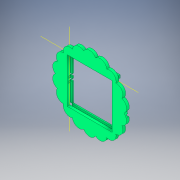
# Autodesk Inventor part: 20_Cube_Insert_CirAp_Wheel
Saved by Autodesk Inventor 2019.4 (Build 234330000, 330)
## iProperties
Created: 2019-10-23
Part Number: 20_Cube_Insert_CirAp_Wheel
Material: Generic
Document SubType Name: Modeling
Designer: marsikovabarbora
Density: 1 g/cm^3
Appearance: Default
Author: marsikovabarbora
Autodesk Inventor part; units mm, degrees
note: some values were not read from the file. Chosen so that the rebuilt part matches the saved one: copy form of "Mirror1".
ref_plane "Work Plane1" through (0, 0, 0) normal (0, 0, 1) x (1, 0, 0)
sketch "Sketch1" plane through (0, 0, 0) normal (0, 0, 1) x (1, 0, 0)
  circle A0 centre (0, 0) radius 20 construction
  line L0 (24.9006, -16.8) -> (24.9006, 16.8) construction
  line L1 (24.9006, 16.8) -> (21.2406, 16.8) construction
  line L2 (21.2406, 16.8) -> (16.8, 21.2406) construction
  line L3 (16.8, 21.2406) -> (16.8, 24.9006) construction
  line L4 (16.8, 24.9006) -> (-16.8, 24.9006) construction
  line L5 (-16.8, 24.9006) -> (-16.8, 21.2406) construction
  line L6 (-16.8, 21.2406) -> (-21.2406, 16.8) construction
  line L7 (-21.2406, 16.8) -> (-24.9006, 16.8) construction
  line L8 (-24.9006, 16.8) -> (-24.9006, -16.8) construction
  line L9 (-24.9006, -16.8) -> (-21.2406, -16.8) construction
  line L10 (-21.2406, -16.8) -> (-16.8, -21.2406) construction
  line L11 (-16.8, -21.2406) -> (-16.8, -24.9006) construction
  line L12 (-16.8, -24.9006) -> (16.8, -24.9006) construction
  line L13 (16.8, -24.9006) -> (16.8, -21.2406) construction
  line L14 (16.8, -21.2406) -> (21.2406, -16.8) construction
  line L15 (21.2406, -16.8) -> (24.9006, -16.8) construction
  line L16 (-36.8547, 0) -> (36.8547, 0) construction
  line L17 (0, -36.4) -> (0, 36.4) construction
  circle A1 centre (0, 0) radius 26
  circle A2 centre (0, 0) radius 22
  point P0 (0, 0)
  dimension "d0" = 52
  dimension "d1" = 44
  constraints: 2 centre point, 2 coincident
  measures "d0" diameter of A1
  measures "d1" diameter of A2
extrude "Extrusion1" add sketch "Sketch1" along normal blind 1.9
sketch "Sketch2" plane through (0, 0, 1.9) normal (0, 0, 1) x (1, 0, 0)
  circle A0 centre (0, 0) radius 22 construction
  circle A1 centre (0, 0) radius 26 construction
  line L0 (0, -36.4197) -> (0, 36.5183) construction
  line L1 (0, 0) -> (-4.5149, 25.605) construction
  line L2 (0, 0) -> (4.5149, 25.605) construction
  arc A2 (0, 26) -> (-4.5149, 25.605) centre (0, 0) ccw
  arc A3 (4.5149, 25.605) -> (0, 26) centre (0, 0) ccw
  arc A4 (4.1452, 23.5087) -> (-4.1452, 23.5087) centre (0, 21.3057) ccw
  line L3 (-4.1452, 23.5087) -> (0, 22) construction
  line L4 (4.1452, 23.5087) -> (0, 22) construction
  line L5 (-4.5149, 25.605) -> (-4.1452, 23.5087)
  line L6 (4.5149, 25.605) -> (4.1452, 23.5087)
  point P0 (0, 26)
  dimension "d62" = 10
  dimension "d63" = 10
  dimension "d65" = 70
  dimension "d66" = 70
  constraints: 12 end point, 8 point on circle, 4 point on line, 3 centre point, 2 collinear, 2 vertical alignment, 1 coincident
  measures "d62" angle of L1 L0
  measures "d63" angle of L2 L0
  measures "d65" angle of L4 L0
  measures "d66" angle of L0 L3
extrude "Extrusion2" cut sketch "Sketch2" against normal up to next
mirror "Mirror1" about plane through (0, 0, 0) normal (1, 0, 0) of "Extrusion2" geometry pattern yes
pattern_circular "Circular Pattern1" count 18 over 360 about axis through (0, 0, -10) along (0, 0, 1) of "Extrusion2", "Mirror1"
sketch "Skizze4" plane through (0, 0, 1.9) normal (0, 0, 1) x (1, 0, 0)
  circle A0 centre (0, 0) radius 22 projected
  line L0 (15.5563, 15.5563) -> (15.5563, -15.5563)
  line L1 (15.5563, -15.5563) -> (-15.5563, -15.5563)
  line L2 (-15.5563, -15.5563) -> (-15.5563, 15.5563)
  line L3 (-15.5563, 15.5563) -> (15.5563, 15.5563)
  arc A1 (-15.5563, 15.5563) -> (-15.5563, -15.5563) centre (0, 0) ccw
  arc A2 (15.5563, 15.5563) -> (-15.5563, 15.5563) centre (0, 0) ccw
  arc A3 (15.5563, -15.5563) -> (15.5563, 15.5563) centre (0, 0) ccw
  arc A4 (-15.5563, -15.5563) -> (15.5563, -15.5563) centre (0, 0) ccw
  point P0 (-15.5563, 0)
  constraints: 8 end point, 8 point on circle, 4 centre point, 2 coincident, 1 horizontal alignment, 1 midpoint, 12 other
extrude "Extrusion4" add sketch "Skizze4" against normal up to surface (1.9 mm away) contours A0 L0 | L3 A0 | A0 L1 | L2 A0
sketch "Skizze5" plane through (0, 0, 0) normal (0, 0, -1) x (-1, 0, 0)
  line L0 (17, 17) -> (17, 15.2314)
  line L1 (17, -17) -> (-17, -17)
  line L2 (-17, -17) -> (-17, 17)
  line L3 (-17, 17) -> (14.1379, 17)
  line L4 (11.6421, 17) -> (14.0421, 17)
  line L5 (17, 15.2314) -> (17, -17)
  line L6 (15.2175, 17) -> (17, 17)
  line L7 (14.1379, 17) -> (15.2175, 17)
  line L8 (15.5563, -15.5563) -> (15.5563, 15.5563) projected
  line L9 (15.5563, 15.5563) -> (-15.5563, 15.5563) projected
  line L10 (-15.5563, 15.5563) -> (-15.5563, -15.5563) projected
  line L11 (-15.5563, -15.5563) -> (15.5563, -15.5563) projected
  arc A0 (-4.1452, 23.5087) -> (-11.9357, 20.6732) centre (-7.287, 20.0208) ccw projected
  arc A1 (4.1452, 23.5087) -> (-4.1452, 23.5087) centre (0, 21.3057) ccw projected
  arc A2 (11.9357, 20.6732) -> (4.1452, 23.5087) centre (7.287, 20.0208) ccw projected
  arc A3 (18.2866, 15.3442) -> (11.9357, 20.6732) centre (13.6951, 16.3211) ccw projected
  arc A4 (22.4318, 8.1645) -> (18.2866, 15.3442) centre (18.4513, 10.6529) ccw projected
  arc A5 (23.8714, 0) -> (22.4318, 8.1645) centre (20.9821, 3.6997) ccw projected
  arc A6 (22.4318, -8.1645) -> (23.8714, 0) centre (20.9821, -3.6997) ccw projected
  arc A7 (18.2866, -15.3442) -> (22.4318, -8.1645) centre (18.4513, -10.6529) ccw projected
  arc A8 (11.9357, -20.6732) -> (18.2866, -15.3442) centre (13.6951, -16.3211) ccw projected
  arc A9 (4.1452, -23.5087) -> (11.9357, -20.6732) centre (7.287, -20.0208) ccw projected
  arc A10 (-4.1452, -23.5087) -> (4.1452, -23.5087) centre (0, -21.3057) ccw projected
  arc A11 (-11.9357, -20.6732) -> (-4.1452, -23.5087) centre (-7.287, -20.0208) ccw projected
  arc A12 (-18.2866, -15.3442) -> (-11.9357, -20.6732) centre (-13.6951, -16.3211) ccw projected
  arc A13 (-22.4318, -8.1645) -> (-18.2866, -15.3442) centre (-18.4513, -10.6529) ccw projected
  arc A14 (-23.8714, 0) -> (-22.4318, -8.1645) centre (-20.9821, -3.6997) ccw projected
  arc A15 (-22.4318, 8.1645) -> (-23.8714, 0) centre (-20.9821, 3.6997) ccw projected
  arc A16 (-18.2866, 15.3442) -> (-22.4318, 8.1645) centre (-18.4513, 10.6529) ccw projected
  arc A17 (-11.9357, 20.6732) -> (-18.2866, 15.3442) centre (-13.6951, 16.3211) ccw projected
  point P0 (0, 0)
  point P1 (0, 0)
  point P2 (0, 17)
  dimension "d26" = 34
  constraints: 16 end point, 2 point on line, 1 coincident, 1 collinear, 1 vertical alignment, 9 other
  measures "d26" distance of L2.end L0.start
ref_plane "Arbeitsebene2" through (7.7782, 15.5563, 0) normal (0, 1, 0) x (1, 0, 0)
sketch "Skizze6" plane through (7.7782, 15.5563, 0) normal (0, 1, 0) x (1, 0, 0)
  line L0 (-26.9158, 0) -> (-26.9158, 0) projected
  line L1 (15.5563, 15.5563) -> (-15.5563, 15.5563)
  line L2 (-23.3345, 0) -> (7.7782, 0) projected
  line L3 (-24.7782, 0) -> (-25.7782, 0)
  line L4 (-24.7782, 1.5) -> (-24.7782, 0)
  line L5 (-24.7782, 19.0476) -> (-24.7782, -5.3913) projected
  line L6 (-23.3345, 0) -> (-27.3072, 0)
  line L7 (-24.7782, 1.5) -> (-23.3782, 1.5)
  line L8 (-23.3782, 1.5) -> (-23.3782, 2.5)
  line L9 (-23.3782, 2.5) -> (-25.2782, 2.5)
  line L10 (-25.2782, 2.5) -> (-25.7782, 0)
  point P0 (-7.7782, 0)
  point P1 (-26.8982, 0)
  dimension "d30" = 1.5
  dimension "d90" = 1
  dimension "d96" = 1.4
  dimension "d97" = 1
  constraints: 16 end point, 2 perpendicular, 1 collinear, 1 horizontal, 1 point on line
  measures "d30" distance of L4.start L3.start
  measures "d90" distance of L3.start L3.end
  measures "d96" distance of L4.start L7.end
  measures "d97" distance between parallel lines of L9 L7
extrude "Extrusion5" add sketch "Skizze6" against normal blind 31
ref_plane "Arbeitsebene4" through (-15.5563, 7.7782, 0) normal (1, 0, 0) x (0, 1, 0)
sketch "Skizze8" plane through (-15.5563, 7.7782, 0) normal (1, 0, 0) x (0, 1, 0)
  line L0 (9.2218, 0) -> (10.2218, 0)
  line L1 (9.2218, -1.5) -> (9.2218, 0)
  line L2 (9.2218, -3.38) -> (9.2218, 2.78) projected
  line L3 (-23.3345, 0) -> (7.7782, 0) projected
  line L4 (7.7782, 0) -> (12.5753, 0)
  line L5 (9.2218, -1.5) -> (7.8218, -1.5)
  line L6 (7.8218, -1.5) -> (7.8218, -2.5)
  line L7 (7.8218, -2.5) -> (9.7218, -2.5)
  line L8 (9.7218, -2.5) -> (10.2218, 0)
  point P0 (-7.7782, 0)
  dimension "d38" = 1.5
  dimension "d92" = 1
  dimension "d94" = 1.4
  dimension "d95" = 1
  constraints: 14 end point, 3 horizontal, 2 perpendicular, 1 collinear
  measures "d38" distance of L1.start L0.start
  measures "d92" distance of L0.start L0.end
  measures "d94" distance of L1.start L5.end
  measures "d95" distance between parallel lines of L5 L7
extrude "Extrusion6" add sketch "Skizze8" along normal blind 32.5
sketch "Skizze12" plane through (0, 0, 0) normal (0, 0, -1) x (-1, 0, 0)
  line L0 (-15.5563, 15.5563) -> (-15.5563, -15.5563) projected
  line L1 (0, 0) -> (34.7318, 0) construction
  line L2 (15.5563, -15.5563) -> (15.5563, 15.5563) construction
  line L3 (15.5563, -0.75) -> (15.5563, -2.25)
  line L4 (15.5563, -2.25) -> (16.5173, -2.25)
  line L5 (15.5563, 0.75) -> (15.5563, -0.75) construction
  arc A0 (25.4469, -2.25) -> (24.6338, -0.75) centre (20.9821, -3.6997) ccw
  line L6 (24.6338, -0.75) -> (22.4775, -0.75)
  line L7 (22.4775, -0.75) -> (17.3303, -0.75)
  arc A1 (24.6338, -0.75) -> (24.6321, -0.7479) centre (20.9821, -3.6997) ccw
  line L8 (16.5173, -2.25) -> (25.4469, -2.25)
  line L9 (17.3303, -0.75) -> (15.5563, -0.75)
  line L10 (15.5563, 0.75) -> (15.5563, 2.25)
  line L11 (15.5563, 2.25) -> (16.5173, 2.25)
  arc A2 (24.6338, 0.75) -> (25.4469, 2.25) centre (20.9821, 3.6997) ccw
  line L12 (24.6338, 0.75) -> (22.4775, 0.75)
  line L13 (22.4775, 0.75) -> (17.3303, 0.75)
  arc A3 (24.6321, 0.7479) -> (24.6338, 0.75) centre (20.9821, 3.6997) ccw
  line L14 (16.5173, 2.25) -> (25.4469, 2.25)
  line L15 (17.3303, 0.75) -> (15.5563, 0.75)
  line L16 (-22.4775, 0.75) -> (-17.3303, 0.75)
  line L17 (-22.4775, -0.75) -> (-17.3303, -0.75)
  line L18 (-16.5173, 2.25) -> (-25.4469, 2.25)
  line L19 (-16.5173, -2.25) -> (-25.4469, -2.25)
  line L20 (-24.6338, 0.75) -> (-22.4775, 0.75)
  line L21 (-24.6338, -0.75) -> (-22.4775, -0.75)
  arc A4 (-24.6321, -0.7479) -> (-24.6338, -0.75) centre (-20.9821, -3.6997) ccw
  arc A5 (-24.6338, -0.75) -> (-25.4469, -2.25) centre (-20.9821, -3.6997) ccw
  arc A6 (-25.4469, 2.25) -> (-24.6338, 0.75) centre (-20.9821, 3.6997) ccw
  arc A7 (-24.6338, 0.75) -> (-24.6321, 0.7479) centre (-20.9821, 3.6997) ccw
  line L22 (-15.5563, 0.75) -> (-15.5563, 2.25)
  line L23 (-15.5563, 2.25) -> (-16.5173, 2.25)
  line L24 (-15.5563, -0.75) -> (-15.5563, 0.75) construction
  line L25 (-17.3303, 0.75) -> (-15.5563, 0.75)
  line L26 (-15.5563, -0.75) -> (-15.5563, -2.25)
  line L27 (-15.5563, -2.25) -> (-16.5173, -2.25)
  line L28 (-17.3303, -0.75) -> (-15.5563, -0.75)
  point P0 (-15.5563, 0)
  point P1 (-15.5563, 0.7473)
  point P2 (-15.5563, -0.7527)
  point P3 (15.5563, 0)
  point P4 (-15.5563, 0)
  dimension "d82" = 1.5
  dimension "d88" = 360
  constraints: 54 end point, 20 point on circle, 8 centre point, 8 symmetric about line, 6 parallel, 3 point on line, 2 midpoint, 2 perpendicular, 1 horizontal, 1 horizontal alignment, 1 vertical, 75 other
  measures "d82" distance between parallel lines of L8 L7
extrude "Extrusion9" cut sketch "Skizze12" against normal blind 1 and the other way blind 3.5
mirror "Spiegeln2" about plane through (0, 0, 0) normal (0, 1, 0) of "Extrusion6"
sketch "Skizze13" plane through (0, 0, 1.9) normal (0, 0, 1) x (1, 0, 0)
  circle A0 centre (0, 0) radius 15.5563
  line L0 (15.5563, 15.5563) -> (15.5563, 2.25) projected
  constraints: 1 centre point, 1 coincident, 1 tangent
body "Solid1"
